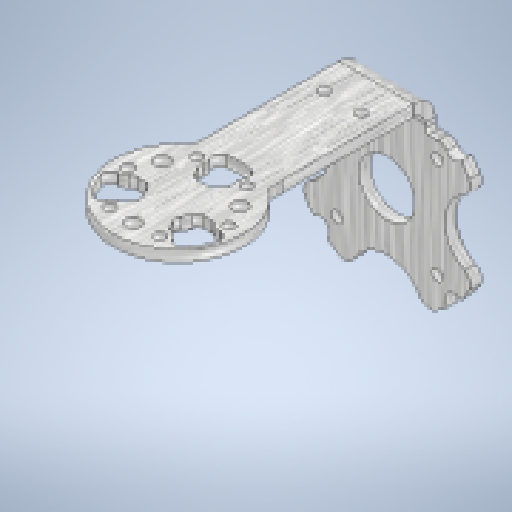
# Autodesk Inventor part: J5_J6_CONNECTOR
Saved by Autodesk Inventor 2025.4 (Build 294407000, 407)
## iProperties
Created: 2026-06-14
Part Number: J5_J6_CONNECTOR
Material: 铝 5052
Document SubType Name: Sheet Metal
Designer: Admin
Density: 2.68 g/cm^3
Sheet Metal Rule: 默认_mm
Appearance: 缎光 - 强拉丝
Mass: 19.4428 g
Surface Area: 67.759 cm^2
Volume: 7.25477 cm^3
Author: Admin
Autodesk Inventor part; units mm, degrees
ref_plane "YZ Plane" through (0, 0, 0) normal (1, 0, 0) x (0, 1, 0)
ref_plane "XZ Plane" through (0, 0, 0) normal (0, 1, 0) x (-1, 0, 0)
ref_plane "XY Plane" through (0, 0, 0) normal (0, 0, 1) x (1, 0, 0)
sketch "草图1" plane through (0, 0, 0) normal (0, 0, 1) x (1, 0, 0)
  arc A0 (19.7736, -16.1014) -> (16.1014, -19.7736) centre (18.0312, -18.0312) ccw
  arc A1 (15.8978, 16.5451) -> (19.7736, 16.1014) centre (18.0312, 18.0312) ccw
  arc A2 (-19.7736, 16.1014) -> (-15.8978, 16.5451) centre (-18.0312, 18.0312) ccw
  arc A3 (-16.1014, -19.7736) -> (-19.7736, -16.1014) centre (-18.0312, -18.0312) ccw
  arc A4 (-20.779, -8.8155) -> (-20.779, 8.8155) centre (-25.5, 0) ccw
  arc A5 (8.8155, -20.779) -> (-8.8155, -20.779) centre (0, -25.5) ccw
  arc A6 (20.779, 8.8155) -> (20.779, -8.8155) centre (25.5, 0) ccw
  arc A7 (-19.7736, 16.1014) -> (-21.9444, 12.9881) centre (0, 0) ccw
  arc A8 (-21.9444, -12.9881) -> (-19.7736, -16.1014) centre (0, 0) ccw
  arc A9 (-16.1014, -19.7736) -> (-12.9881, -21.9444) centre (0, 0) ccw
  arc A10 (12.9881, -21.9444) -> (16.1014, -19.7736) centre (0, 0) ccw
  arc A11 (19.7736, -16.1014) -> (21.9444, -12.9881) centre (0, 0) ccw
  arc A12 (21.9444, 12.9881) -> (19.7736, 16.1014) centre (0, 0) ccw
  arc A13 (-20.779, -8.8155) -> (-21.9444, -12.9881) centre (-19.3627, -11.4601) ccw
  arc A14 (-12.9881, -21.9444) -> (-8.8155, -20.779) centre (-11.4601, -19.3627) ccw
  arc A15 (8.8155, -20.779) -> (12.9881, -21.9444) centre (11.4601, -19.3627) ccw
  arc A16 (21.9444, -12.9881) -> (20.779, -8.8155) centre (19.3627, -11.4601) ccw
  arc A17 (20.779, 8.8155) -> (21.9444, 12.9881) centre (19.3627, 11.4601) ccw
  arc A18 (-21.9444, 12.9881) -> (-20.779, 8.8155) centre (-19.3627, 11.4601) ccw
  circle A19 centre (-13.435, -13.435) radius 1.5
  circle A20 centre (-13.435, 13.435) radius 1.5
  circle A21 centre (13.435, -13.435) radius 1.5
  circle A22 centre (13.435, 13.435) radius 1.5
  line L0 (0, 32.7) -> (0, -35.2)
  line L1 (-35.7, 0) -> (35.7, 0)
  line L2 (-10, 20) -> (-10, 18.8304)
  line L3 (10, 20) -> (10, 18.8304)
  line L4 (13.4361, 17.8304) -> (11, 17.8304)
  line L5 (-11, 17.8304) -> (-13.4361, 17.8304)
  arc A23 (-13.4361, 17.8304) -> (-15.8978, 16.5451) centre (-13.4361, 14.8304) ccw
  arc A24 (15.8978, 16.5451) -> (13.4361, 17.8304) centre (13.4361, 14.8304) ccw
  arc A25 (-11, 17.8304) -> (-10, 18.8304) centre (-11, 18.8304) ccw
  arc A26 (10, 18.8304) -> (11, 17.8304) centre (11, 18.8304) ccw
  line L6 (-10, 20) -> (-10, 23)
  line L7 (-10, 23) -> (10, 23)
  line L8 (10, 23) -> (10, 20)
  point P0 (0, 0)
  point P1 (15.439, 17.8304)
  point P2 (-15.439, 17.8304)
  dimension "d0" = 20
  dimension "d1" = 20
  dimension "d2" = 20
  dimension "d3" = 3
  dimension "d4" = 3
  dimension "d5" = 3
  dimension "d6" = 3
  dimension "d7" = 3
  dimension "d11" = 3
  dimension "d12" = 1
  dimension "d14" = 3
  measures "d0" diameter of A4
  measures "d1" diameter of A5
  measures "d2" diameter of A6
  measures "d3" radius of A13
  measures "d4" diameter of A19
  measures "d5" diameter of A20
  measures "d6" diameter of A21
  measures "d7" diameter of A22
  measures "d11" radius of A23
  measures "d12" radius of A25
  measures "d14" distance of L7.end L3.start
extrude "平板1" add sketch "草图1" along normal blind 3
sketch "草图2" plane through (-10, 26, 0) normal (0, -1, 0) x (1, 0, 0)
  line L0 (20, 0) -> (0, 0)
  line L1 (0, 0) -> (0, 41.25)
  line L2 (0, 41.25) -> (20, 41.25)
  line L3 (20, 41.25) -> (20, 0)
  constraints: 8 end point
bend "折弯1"
corner "拐角1"
edge flange "凸缘1" height 41.25 angle 90 thickness 3 bend radius 3 thickness toward (0, -1, 0) relief tear relief width 3 relief depth 1.5 edges at (0, 23, 3) wall of the first edge with corners at (10, 26, 0) (-10, 26, 0) (-10, 26, 41.25) (10, 26, 41.25)
sketch "草图4" plane through (-10, 26, 41.25) normal (0, 1, 0) x (1, 0, 0)
  arc A0 (0, -3.5106) -> (20.1459, -3.6142) centre (10, -17.75) ccw
  circle A1 centre (20.5222, -11.675) radius 2
  circle A2 centre (-0.5222, -11.675) radius 2
  circle A3 centre (10, -29.9) radius 2
  arc A4 (13.408, -1.6058) -> (6.592, -1.6058) centre (10, -17.75) ccw
  arc A5 (14.727, -4.5627) -> (13.408, -1.6058) centre (12.9949, -3.5627) ccw
  line L0 (14.5849, -4.8087) -> (14.727, -4.5627)
  arc A6 (14.5849, -4.8087) -> (14.3749, -6.8391) centre (16.75, -6.0587) ccw
  arc A7 (14.2069, -8.4634) -> (14.3749, -6.8391) centre (12.4749, -7.4634) ccw
  line L1 (13.1105, -10.3625) -> (14.2069, -8.4634)
  arc A8 (11.0541, -11.336) -> (13.1105, -10.3625) centre (11.3784, -9.3625) ccw
  arc A9 (11.0541, -11.336) -> (8.9459, -11.336) centre (10, -17.75) ccw
  arc A10 (6.8895, -10.3625) -> (8.9459, -11.336) centre (8.6216, -9.3625) ccw
  line L2 (5.7931, -8.4634) -> (6.8895, -10.3625)
  arc A11 (5.6251, -6.8391) -> (5.7931, -8.4634) centre (7.5251, -7.4634) ccw
  arc A12 (5.6251, -6.8391) -> (5.4151, -4.8087) centre (3.25, -6.0587) ccw
  line L3 (5.273, -4.5627) -> (5.4151, -4.8087)
  arc A13 (6.592, -1.6058) -> (5.273, -4.5627) centre (7.0051, -3.5627) ccw
  arc A14 (22.2773, -28.7735) -> (25.6853, -22.8707) centre (10, -17.75) ccw
  arc A15 (19.0571, -28.4373) -> (22.2773, -28.7735) centre (20.7891, -27.4373) ccw
  line L4 (18.9151, -28.1913) -> (19.0571, -28.4373)
  arc A16 (18.9151, -28.1913) -> (17.2617, -26.9943) centre (16.75, -29.4413) ccw
  arc A17 (15.939, -26.0366) -> (17.2617, -26.9943) centre (17.671, -25.0366) ccw
  line L5 (14.8425, -24.1375) -> (15.939, -26.0366)
  arc A18 (15.0276, -21.8698) -> (14.8425, -24.1375) centre (16.5746, -23.1375) ccw
  arc A19 (15.0276, -21.8698) -> (16.0817, -20.0441) centre (10, -17.75) ccw
  arc A20 (17.953, -18.75) -> (16.0817, -20.0441) centre (17.953, -20.75) ccw
  line L6 (17.953, -18.75) -> (20.1459, -18.75)
  arc A21 (21.6366, -19.4167) -> (20.1459, -18.75) centre (20.1459, -20.75) ccw
  arc A22 (21.6366, -19.4167) -> (23.5, -20.25) centre (23.5, -17.75) ccw
  line L7 (23.5, -20.25) -> (23.784, -20.25)
  arc A23 (25.6853, -22.8707) -> (23.784, -20.25) centre (23.784, -22.25) ccw
  arc A24 (-2.2773, -28.7735) -> (0.9429, -28.4373) centre (-0.7891, -27.4373) ccw
  arc A25 (-5.6853, -22.8707) -> (-2.2773, -28.7735) centre (10, -17.75) ccw
  arc A26 (-3.784, -20.25) -> (-5.6853, -22.8707) centre (-3.784, -22.25) ccw
  line L8 (-3.784, -20.25) -> (-3.5, -20.25)
  arc A27 (-3.5, -20.25) -> (-1.6366, -19.4167) centre (-3.5, -17.75) ccw
  arc A28 (-0.1459, -18.75) -> (-1.6366, -19.4167) centre (-0.1459, -20.75) ccw
  line L9 (-0.1459, -18.75) -> (2.047, -18.75)
  arc A29 (3.9183, -20.0441) -> (2.047, -18.75) centre (2.047, -20.75) ccw
  arc A30 (3.9183, -20.0441) -> (4.9724, -21.8698) centre (10, -17.75) ccw
  arc A31 (5.1575, -24.1375) -> (4.9724, -21.8698) centre (3.4254, -23.1375) ccw
  line L10 (4.061, -26.0366) -> (5.1575, -24.1375)
  arc A32 (2.7383, -26.9943) -> (4.061, -26.0366) centre (2.329, -25.0366) ccw
  arc A33 (2.7383, -26.9943) -> (1.0849, -28.1913) centre (3.25, -29.4413) ccw
  line L11 (0.9429, -28.4373) -> (1.0849, -28.1913)
  circle A34 centre (10, -17.75) radius 4.75
  line L12 (0, 35.25) -> (0, 0)
  line L13 (0, 0) -> (20.1459, 0)
  line L14 (0, -3.5106) -> (0, 0)
  line L15 (20.1459, 0) -> (20.1459, -3.6142)
  circle A35 centre (16.75, -6.0587) radius 1.5
  circle A36 centre (23.5, -17.75) radius 1.5
  circle A37 centre (-3.5, -17.75) radius 1.5
  circle A38 centre (3.25, -6.0587) radius 1.5
  circle A39 centre (16.75, -29.4413) radius 1.5
  circle A40 centre (3.25, -29.4413) radius 1.5
  point P0 (10, 41.25)
  dimension "d52" = 3
  dimension "d53" = 3
  dimension "d56" = 360
  measures "d52" diameter of A35
  measures "d53" diameter of A36
sheet face with bend "平板2" sketch "草图4" thickness 3 toward (0, -1, 0) bend radius 3
bend "折弯2"
sketch "草图7" plane through (-10, 26, 6) normal (0, 1, 0) x (1, 0, 0)
  line L0 (20, 0) -> (0, 0) projected
  line L1 (0, -38.7606) -> (0, 0) projected
  point P0 (10, 6)
  point P1 (15, -9)
  point P2 (5, -9)
  point P3 (0, -28.7606)
  point P4 (0, -35.25)
  dimension "d39" = 9
  dimension "d40" = 10
  dimension "d41" = 5
  constraints: 1 horizontal alignment
  measures "d39" distance from line of L0 point (15, -9)
  measures "d40" distance of point (5, -9) point (15, -9)
  measures "d41" distance from line of L1 point (5, -9)
hole "孔2" at (5, 26, 15) at (-5, 26, 15) direction (0, -1, 0) diameter 3 end through all
sketch "草图8" plane through (0, 0, 3) normal (0, 0, 1) x (1, 0, 0)
  circle A0 centre (0, 0) radius 7.5
  dimension "d49" = 15
  constraints: 1 centre point, 1 coincident
  measures "d49" diameter of A0
extrude "拉伸2" cut sketch "草图8" against normal blind 10
equation "\"d13\" = 厚度"
equation "\"d15\" = 折弯释压宽度"
equation "\"d16\" = 折弯释压深度"
equation "\"d17\" = 最小余量"
equation "\"d18\" = 过渡半径"
equation "\"d21\" = 折弯半径"
equation "\"d22\" = 拐角释压尺寸"
equation "\"d23\" = 间隙大小"
equation "\"d24\" = Jacobi半径尺寸"
equation "\"d25\" = 折弯半径"
equation "\"d26\" = 折弯释压宽度"
equation "\"d28\" = 最小余量"
equation "\"d27\" = 折弯释压深度"
equation "\"d29\" = 过渡半径"
equation "\"折弯半径\" = 厚度"
equation "\"折弯释压宽度\" = 厚度"
equation "\"折弯释压深度\" = 0.5 * 厚度"
equation "\"拐角释压尺寸\" = 4 * 厚度"
equation "\"最小余量\" = 2 * 厚度"
equation "\"过渡半径\" = 折弯半径"
equation "\"Jacobi半径尺寸\" = 折弯半径"
equation "\"间隙大小\" = 厚度"
equation "\"厚度\" = 3"
